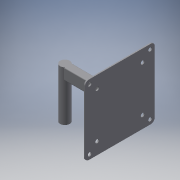
# Autodesk Inventor part: MonitorMount
Saved by Autodesk Inventor 2018 (Build 220105000, 105)
## iProperties
Created: 2004-11-28
Document SubType Name: Modeling
Designer: Autodesk, Inc.
Manufacturer: Standard
Standards Organization: Custom
Description: SWING ARM MONITOR MOUNT
Mass: 79.9167 g
Surface Area: 366.222 cm^2
Volume: 79.9167 cm^3
Density: 1 g/cm^3
Material: Generic
Appearance: Default
CAGE: 1LJX3
Dept. ID: Product Design
Description #2: ---
Finish #1: ---
Finish #2: ---
Material ID: ---
Project Number: ---
Author: Autodesk, Inc.
Autodesk Inventor part; units mm, degrees
ref_plane "YZ Plane" through (0, 0, 0) normal (1, 0, 0) x (0, 1, 0)
ref_plane "XZ Plane" through (0, 0, 0) normal (0, 1, 0) x (-1, 0, 0)
sketch "Sketch1" plane through (0, 0, 0) normal (0, 0, 1) x (1, 0, 0)
  line L0 (0, 41.275) -> (7.9375, 41.275)
  line L1 (7.9375, 41.275) -> (7.9375, -41.275)
  line L2 (7.9375, -41.275) -> (0, -41.275)
  line L3 (0, -41.275) -> (0, 41.275)
  point P0 (0, 0)
  point P1 (0, 0)
  dimension "d0" = 15.875
  dimension "d1" = 82.55
  constraints: 8 end point, 2 midpoint, 2 parallel, 1 coincident, 1 horizontal, 1 perpendicular
  measures "d0" diameter of L1 L3
  measures "d1" distance between parallel lines of L2 L0
revolve "Revolution1" add sketch "Sketch1" angle 360 about axis through (0, -41.275, 0) along (0, 1, 0)
sketch "Sketch2" plane through (0, 0, 0) normal (0, 0, 1) x (1, 0, 0)
  line L0 (-7.9375, 41.275) -> (7.9375, 41.275) projected
  line L1 (7.9375, 41.275) -> (7.9375, -41.275) projected
  line L2 (0, -58.42) -> (0, 61.595) projected
  line L3 (0, 41.275) -> (38.1, 41.275)
  line L4 (38.1, 41.275) -> (38.1, 22.225)
  line L5 (38.1, 22.225) -> (0, 22.225)
  line L6 (0, 22.225) -> (0, 41.275)
  line L7 (38.1, 41.275) -> (88.9, 44.45)
  line L8 (88.9, 44.45) -> (88.9, 19.05)
  line L9 (88.9, 19.05) -> (38.1, 22.225)
  line L10 (88.9, 31.75) -> (38.1, 31.75) construction
  dimension "d3" = 19.05
  dimension "d4" = 38.1
  dimension "d5" = 25.4
  dimension "d6" = 88.9
  constraints: 16 end point, 3 midpoint, 3 parallel, 2 perpendicular, 1 horizontal, 1 point on line, 1 other
  measures "d3" distance between parallel lines of L3 L5
  measures "d4" distance between parallel lines of L2 L4
  measures "d5" distance of L7.end L8.end
  measures "d6" distance between parallel lines of L2 L8
extrude "Extrusion1" add sketch "Sketch2" along normal mid plane 12.7
sketch "Sketch4" plane through (88.9, 19.05, 6.35) normal (1, 0, 0) x (0, 0, -1)
  line L0 (0, 25.4) -> (0, 0) projected
  line L1 (12.7, 0) -> (0, 0) projected
  line L2 (12.7, 0) -> (12.7, 25.4) projected
  line L3 (12.7, 25.4) -> (0, 25.4) projected
  line L4 (-44.831, 70.231) -> (57.531, 70.231)
  line L5 (63.881, 63.881) -> (63.881, -38.481)
  line L6 (57.531, -44.831) -> (-44.831, -44.831)
  line L7 (-51.181, -38.481) -> (-51.181, 63.881)
  arc A0 (-44.831, 70.231) -> (-51.181, 63.881) centre (-44.831, 63.881) ccw
  arc A1 (63.881, 63.881) -> (57.531, 70.231) centre (57.531, 63.881) ccw
  arc A2 (57.531, -44.831) -> (63.881, -38.481) centre (57.531, -38.481) ccw
  arc A3 (-51.181, -38.481) -> (-44.831, -44.831) centre (-44.831, -38.481) ccw
  point P0 (-51.181, 70.231)
  point P1 (63.881, 70.231)
  point P2 (-51.181, 12.7)
  point P3 (0, 12.7)
  point P4 (6.35, 70.231)
  point P5 (6.35, 25.4)
  dimension "d9" = 115.062
  dimension "d10" = 6.35
  constraints: 8 end point, 8 point on circle, 8 tangent, 4 centre point, 4 midpoint, 4 point on line, 3 equal radius, 2 parallel, 2 perpendicular, 1 horizontal, 1 horizontal alignment, 1 vertical alignment
  measures "d9" distance of point (-51.181, 70.231) point (63.881, 70.231)
  measures "d10" radius of A0
extrude "Extrusion2" add sketch "Sketch4" along normal blind 1.905 contours L3 L2 L1 L0 | L4 A1 L5 A2 L6 A3 L7 A0
sketch "Sketch5" plane through (88.9, 19.05, 6.35) normal (-1, 0, 0) x (0, 0, 1)
  arc A0 (51.181, 63.881) -> (44.831, 70.231) centre (44.831, 63.881) ccw projected
  line L0 (-57.531, 70.231) -> (44.831, 70.231) projected
  arc A1 (-57.531, 70.231) -> (-63.881, 63.881) centre (-57.531, 63.881) ccw projected
  line L1 (-63.881, -38.481) -> (-63.881, 63.881) projected
  arc A2 (-63.881, -38.481) -> (-57.531, -44.831) centre (-57.531, -38.481) ccw projected
  line L2 (44.831, -44.831) -> (-57.531, -44.831) projected
  arc A3 (44.831, -44.831) -> (51.181, -38.481) centre (44.831, -38.481) ccw projected
  line L3 (51.181, 63.881) -> (51.181, -38.481) projected
  line L4 (-12.7, 0) -> (-12.7, 25.4) projected
  line L5 (-12.7, 25.4) -> (0, 25.4) projected
  line L6 (0, 25.4) -> (0, 0) projected
  line L7 (-12.7, 0) -> (0, 0) projected
  line L8 (-23.8125, 44.45) -> (11.1125, 44.45)
  line L9 (17.4625, 38.1) -> (17.4625, -12.7)
  line L10 (11.1125, -19.05) -> (-23.8125, -19.05)
  line L11 (-30.1625, -12.7) -> (-30.1625, 38.1)
  arc A4 (-23.8125, 44.45) -> (-30.1625, 38.1) centre (-23.8125, 38.1) ccw
  arc A5 (17.4625, 38.1) -> (11.1125, 44.45) centre (11.1125, 38.1) ccw
  arc A6 (11.1125, -19.05) -> (17.4625, -12.7) centre (11.1125, -12.7) ccw
  arc A7 (-30.1625, -12.7) -> (-23.8125, -19.05) centre (-23.8125, -12.7) ccw
  line L12 (-12.7, 25.4) -> (0, 25.4) projected
  line L13 (-12.7, 0) -> (-12.7, 25.4) projected
  point P0 (-6.35, 44.45)
  point P1 (-6.35, 25.4)
  point P2 (-30.1625, 12.7)
  point P3 (-12.7, 12.7)
  dimension "d13" = 6.35
  dimension "d14" = 63.5
  dimension "d15" = 47.625
  constraints: 8 end point, 8 point on circle, 8 tangent, 4 centre point, 4 midpoint, 3 equal radius, 2 parallel, 1 horizontal, 1 horizontal alignment, 1 perpendicular, 1 vertical alignment
  measures "d13" radius of A4
  measures "d14" distance between parallel lines of L10 L8
  measures "d15" distance between parallel lines of L9 L11
extrude "Extrusion3" add sketch "Sketch5" along normal blind 6.35 fills toward (-6.35, 44.4) open curves L8 A5 L9 A6 L10 A7 L11 A4
fillet "Fillet1" radius 3.175 20 edges at (82.55, 31.75, -6.35) (82.55, 44.0531, 0) (82.55, 31.75, 6.35) (82.55, 19.4469, 0) (82.55, 61.6401, 21.9526) (88.9, 61.6401, 21.9526) (82.55, 31.75, 23.8125) (82.55, 1.8599, 21.9526) (82.55, 0, 0) (82.55, 1.8599, -21.9526) (82.55, 31.75, -23.8125) (82.55, 61.6401, -21.9526) (82.55, 63.5, 0) (88.9, 31.75, 23.8125) (88.9, 1.8599, 21.9526) (88.9, 0, 0) (88.9, 1.8599, -21.9526) (88.9, 31.75, -23.8125) (88.9, 61.6401, -21.9526) (88.9, 63.5, 0)
fillet "Fillet2" radius 1.5875 18 edges at (58.7376, 42.5648, -6.35) (38.1, 41.275, 0) (58.7376, 42.5648, 6.35) (58.7376, 20.9352, -6.35) (21.4313, 22.225, -6.35) (21.4312, 41.275, -6.35) (21.4312, 41.275, 6.35) (21.4313, 22.225, 6.35) (58.7376, 20.9352, 6.35) (38.1, 22.225, 0) (79.4742, 43.8609, -6.3515) (81.6891, 44.8619, -7.3511) (79.4742, 43.8609, 6.3515) (81.6891, 44.8619, 7.3511) (79.4742, 19.6391, -6.3515) (81.6891, 18.6381, -7.3511) (79.4742, 19.6391, 6.3515) (81.6891, 18.6381, 7.3511)
sketch "Sketch6" plane through (90.805, 19.05, 6.35) normal (1, 0, 0) x (0, 0, -1)
  line L0 (-44.831, 70.231) -> (57.531, 70.231) construction
  arc A0 (-44.831, 70.231) -> (-51.181, 63.881) centre (-44.831, 63.881) ccw construction
  line L1 (-51.181, -38.481) -> (-51.181, 63.881) construction
  arc A1 (-51.181, -38.481) -> (-44.831, -44.831) centre (-44.831, -38.481) ccw construction
  line L2 (57.531, -44.831) -> (-44.831, -44.831) construction
  arc A2 (57.531, -44.831) -> (63.881, -38.481) centre (57.531, -38.481) ccw construction
  line L3 (63.881, 63.881) -> (63.881, -38.481) construction
  arc A3 (63.881, 63.881) -> (57.531, 70.231) centre (57.531, 63.881) ccw construction
  line L4 (6.35, 70.231) -> (6.35, -44.831) construction
  line L5 (-51.181, 12.7) -> (63.881, 12.7) construction
  circle A4 centre (-43.65, -37.3) radius 3
  circle A5 centre (-31.15, -24.8) radius 3
  line L6 (6.35, 12.7) -> (-44.831, -38.481) construction
  dimension "d21" = 75
  dimension "d22" = 100
  dimension "d23" = 6
  constraints: 6 end point, 5 midpoint, 2 centre point, 2 point on line, 1 equal radius
  measures "d21" diameter of A5.centre L4
  measures "d22" diameter of A4.centre L4
  measures "d23" diameter of A5
extrude "Extrusion4" cut sketch "Sketch6" against normal through all
ref_plane "Work Plane1" through (88.9, 31.75, 51.181) normal (0, 1, 0) x (1, 0, 0)
mirror "Mirror1" about plane through (88.9, 31.75, 51.181) normal (0, 1, 0) of "Extrusion4"
mirror "Mirror2" about plane through (0, 0, 0) normal (0, 0, 1) of "Extrusion4", "Mirror1"
body "Solid1"
